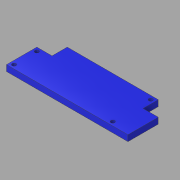
# Autodesk Inventor part: STARduino Mount
Saved by Autodesk Inventor 2017 (Build 210142000, 142)
## iProperties
Created: 2017-01-17
Part Number: STARduino Mount
Material: Polystyrene, High Impact
Document SubType Name: Modeling
Designer: qupec
Density: 1.022 g/cm^3
Appearance: Smooth - White
Author: qupec
Autodesk Inventor part; units mm, degrees
ref_plane "YZ Plane" through (0, 0, 0) normal (1, 0, 0) x (0, 1, 0)
ref_plane "XZ Plane" through (0, 0, 0) normal (0, 1, 0) x (-1, 0, 0)
ref_plane "XY Plane" through (0, 0, 0) normal (0, 0, 1) x (1, 0, 0)
sketch "Sketch1" plane through (0, 0, 0) normal (0, 1, 0) x (-1, 0, 0)
  line L0 (50.8, 19.05) -> (-50.8, 19.05)
  line L1 (-50.8, 19.05) -> (-50.8, -6.35)
  line L2 (50.8, -6.35) -> (50.8, 19.05)
  line L3 (-38.1, -6.35) -> (-38.1, -19.05)
  line L4 (-38.1, -19.05) -> (38.1, -19.05)
  line L5 (38.1, -19.05) -> (38.1, -6.35)
  line L6 (-50.8, -6.35) -> (-38.1, -6.35)
  line L7 (38.1, -6.35) -> (50.8, -6.35)
  point P0 (0, 0)
  dimension "d0" = 25.4
  dimension "d1" = 25.4
  dimension "d2" = 12.7
  dimension "d3" = 12.7
  dimension "d4" = 101.6
  dimension "d5" = 76.2
  dimension "d6" = 12.7
  dimension "d7" = 12.7
  dimension "d8" = 50.8
  dimension "d9" = 38.1
  dimension "d10" = 19.05
  dimension "d11" = 12.7
  constraints: 16 end point, 4 parallel, 1 horizontal, 1 perpendicular
  measures "d0" distance between parallel lines of L7 L0
  measures "d1" distance between parallel lines of L0 L6
  measures "d2" distance between parallel lines of L4 L7
  measures "d3" distance between parallel lines of L4 L6
  measures "d4" distance of L0.start L0.end
  measures "d5" distance of L3.end L4.end
  measures "d6" distance of L5.end L2.start
  measures "d7" distance of L1.end L3.start
  measures "d8" distance from line of point (0, 0) L2
  measures "d9" distance between parallel lines of L4 L0
  measures "d10" distance from line of L0 point (0, 0)
  measures "d11" distance of L4.end L5.end
extrude "Extrusion1" add sketch "Sketch1" along normal blind 5
sketch "Sketch2" plane through (0, 5, 0) normal (0, 1, 0) x (1, 0, 0)
  circle A0 centre (-47.625, -15.875) radius 1.5875
  circle A1 centre (-47.625, 3.175) radius 1.5875
  circle A2 centre (34.925, 15.875) radius 1.5875
  circle A3 centre (34.925, -15.875) radius 1.5875
  line L0 (38.1, 6.35) -> (38.1, 19.05) projected
  line L1 (-50.8, 6.35) -> (-50.8, -19.05) projected
  line L2 (-50.8, -19.05) -> (50.8, -19.05) projected
  line L3 (-38.1, 6.35) -> (-50.8, 6.35) projected
  line L4 (38.1, 19.05) -> (-38.1, 19.05) projected
  point P0 (0, 0)
  dimension "d14" = 3.175
  dimension "d15" = 3.175
  dimension "d16" = 3.175
  dimension "d17" = 3.175
  dimension "d18" = 3.175
  dimension "d19" = 3.175
  dimension "d20" = 3.175
  dimension "d21" = 3.175
  dimension "d22" = 3.175
  dimension "d23" = 3.175
  dimension "d24" = 3.175
  dimension "d25" = 3.175
  constraints: 4 centre point
  measures "d14" distance from line of L0 A3.centre
  measures "d15" diameter of A3
  measures "d16" diameter of A2
  measures "d17" diameter of A0
  measures "d18" diameter of A1
  measures "d19" distance from line of L1 A0.centre
  measures "d20" distance from line of L2 A3.centre
  measures "d21" distance from line of L2 A0.centre
  measures "d22" distance from line of L3 A1.centre
  measures "d23" distance from line of L4 A2.centre
  measures "d24" distance from line of L0 A2.centre
  measures "d25" distance from line of L1 A1.centre
extrude "Extrusion2" cut sketch "Sketch2" against normal through all
equation "\"d1\" = d0"
equation "\"d8\" = 0.5 * d4"
equation "\"d10\" = 0.5 * d9"
equation "\"d16\" = d15"
equation "\"d17\" = d15"
equation "\"d18\" = d15"
equation "\"d19\" = d14"
equation "\"d21\" = d20"
equation "\"d22\" = d20"
equation "\"d23\" = d20"
equation "\"d24\" = d14"
equation "\"d25\" = d14"
body "Solid1"
